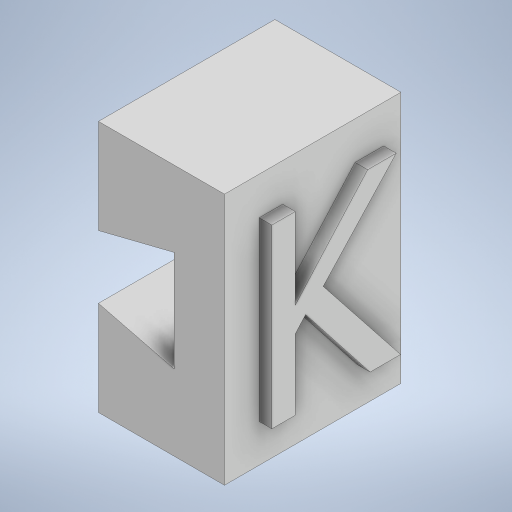
# Autodesk Inventor part: literka
Saved by Autodesk Inventor 2023 (Build 270158000, 158)
## iProperties
Created: 2024-04-25
Part Number: literka
Material: Ogólny
Document SubType Name: Modeling
Designer: Kamil
Density: 1 g/cm^3
Appearance: Domyślna
Author: Kamil
Autodesk Inventor part; units mm, degrees
ref_plane "YZ Plane" through (0, 0, 0) normal (1, 0, 0) x (0, 1, 0)
ref_plane "XZ Plane" through (0, 0, 0) normal (0, 1, 0) x (-1, 0, 0)
ref_plane "XY Plane" through (0, 0, 0) normal (0, 0, 1) x (1, 0, 0)
sketch "Szkic1" plane through (0, 0, 0) normal (1, 0, 0) x (0, 1, 0)
  line L0 (6, 4) -> (-4, 4)
  line L1 (-4, 4) -> (-4, -3)
  line L2 (-4, -3) -> (6, -3)
  line L3 (6, -3) -> (6, 4)
  point P0 (0, 0)
  dimension "d0" = 10
  dimension "d1" = 7
  constraints: 8 end point, 2 parallel, 1 horizontal, 1 perpendicular
  measures "d0" distance of L2.end L1.end
  measures "d1" distance of L1.end L0.end
extrude "Wyciągnięcie proste1" add sketch "Szkic1" against normal blind 5
sketch "Szkic2" plane through (0, 0, 0) normal (1, 0, 0) x (0, 0, -1)
  line L0 (-4, -4) -> (3, -4) projected
  line L1 (3, -4) -> (3, 6) projected
  line L2 (3, 6) -> (-4, 6) projected
  line L3 (-4, 6) -> (-4, -4) projected
  line L4 (-4, 6) -> (3, 6) construction
  line L5 (3, 6) -> (3, -4) construction
  line L6 (3, -4) -> (-4, -4) construction
  line L7 (-4, -4) -> (-4, 6) construction
  line L8 (2.4838, -2.5) -> (1.2755, -2.5)
  line L9 (1.2755, -2.5) -> (-1.2828, 0.7561)
  line L10 (-1.2828, 0.7561) -> (-1.6912, 0.2966)
  line L11 (-1.6912, 0.2966) -> (-1.6912, -2.5)
  line L12 (-1.6912, -2.5) -> (-2.6216, -2.5)
  line L13 (-2.6216, -2.5) -> (-2.6216, 4.5)
  line L14 (-2.6216, 4.5) -> (-1.6912, 4.5)
  line L15 (-1.6912, 4.5) -> (-1.6912, 1.2836)
  line L16 (-1.6912, 1.2836) -> (1.1791, 4.5)
  line L17 (1.1791, 4.5) -> (2.3136, 4.5)
  line L18 (2.3136, 4.5) -> (-0.5851, 1.3744)
  line L19 (-0.5851, 1.3744) -> (2.4838, -2.5)
  point P0 (0, 0)
  point P1 (-0.5, 6)
  point P2 (-0.5, 6)
  point P3 (3, 1)
  point P4 (3, 1)
  dimension "d4" = 10
  dimension "d5" = 7
  constraints: 4 midpoint, 2 coincident, 2 other
  measures "d4" distance of L4.end L5.end
  measures "d5" distance of L5.end L6.end
extrude "Wyciągnięcie proste2" add sketch "Szkic2" along normal blind 0.5 contours L8 L9 L10 L11 L12 L13 L14 L15 L16 L17 L18 L19
sketch "Szkic3" plane through (0, -4, -3) normal (0, 0, -1) x (-1, 0, 0)
  line L0 (2, 7) -> (2, 3)
  line L1 (2, 3) -> (5, 3.75)
  line L2 (2, 7) -> (5, 6.25)
  line L3 (5, 6.25) -> (5, 3.75)
  line L4 (5, 10) -> (5, 0) projected
  point P0 (0, 4)
  point P1 (5, 5)
  point P2 (5, 5)
  point P3 (2, 5)
  point P4 (5, 5)
  dimension "d8" = 4
  dimension "d12" = 3
  dimension "d13" = 2.5
  constraints: 10 end point, 4 midpoint, 2 coincident, 1 horizontal alignment, 1 parallel, 1 vertical
  measures "d8" distance of L0.start L0.end
  measures "d12" distance between parallel lines of L3 L0
  measures "d13" distance of L2.end L1.end
extrude "Wyciągnięcie proste3" cut sketch "Szkic3" against normal blind 10
